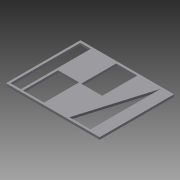
# Autodesk Inventor part: Molecule Chopper
Saved by Autodesk Inventor 2015 (Build 190159000, 159)
## iProperties
Created: 2014-07-07
Part Number: Molecule Chopper
Material: Generic
Document SubType Name: Modeling
Designer: I Rabey
Density: 1 g/cm^3
Appearance: Default
Author: I Rabey
Autodesk Inventor part; units mm, degrees
ref_plane "YZ Plane" through (0, 0, 0) normal (1, 0, 0) x (0, 1, 0)
ref_plane "XZ Plane" through (0, 0, 0) normal (0, 1, 0) x (-1, 0, 0)
ref_plane "XY Plane" through (0, 0, 0) normal (0, 0, 1) x (1, 0, 0)
sketch "Sketch1" plane through (0, 0, 0) normal (0, 1, 0) x (-1, 0, 0)
  line L0 (-42.5, 33.75) -> (42.5, 33.75)
  line L1 (42.5, 33.75) -> (42.5, -33.75)
  line L2 (42.5, -33.75) -> (-42.5, -33.75)
  line L3 (-42.5, -33.75) -> (-42.5, 33.75)
  line L4 (-42.5, 33.75) -> (42.5, -33.75) construction
  line L5 (42.5, 33.75) -> (-42.5, -33.75) construction
  line L6 (60.5225, 31.75) -> (41.4725, 31.75)
  line L7 (40.5, 31.75) -> (30.9975, 31.75)
  line L8 (30.9975, 31.75) -> (30.9975, -31.75)
  line L9 (30.9975, -31.75) -> (40.5, -31.75)
  line L10 (40.5, -31.75) -> (40.5, 31.75)
  line L11 (40.5, 31.75) -> (30.9975, -31.75) construction
  line L12 (30.9975, 31.75) -> (40.5, -31.75) construction
  line L13 (28.9975, 31.75) -> (9.9475, 31.75)
  line L14 (9.9475, 31.75) -> (9.9475, 0)
  line L15 (9.9475, 0) -> (28.9975, 0)
  line L16 (28.9975, 0) -> (28.9975, 31.75)
  line L17 (7.9475, 0) -> (-11.1025, 0)
  line L18 (-11.1025, 0) -> (-11.1025, -31.75)
  line L19 (-11.1025, -31.75) -> (7.9475, -31.75)
  line L20 (7.9475, -31.75) -> (7.9475, 0)
  line L21 (-13.1025, 31.75) -> (-32.1525, 31.75)
  line L22 (-32.1525, 31.75) -> (-32.1525, -31.75)
  line L23 (-32.1525, -31.75) -> (-13.1025, 31.75)
  point P0 (0, 0)
  point P1 (35.7488, 0)
  dimension "d0" = 85
  dimension "d1" = 67.5
  dimension "d5" = 9.5025
  dimension "d6" = 63.5
  dimension "d9" = 19.05
  dimension "d10" = 31.75
  dimension "d11" = 0
  dimension "d12" = 2
  dimension "d13" = 19.05
  dimension "d14" = 31.75
  dimension "d15" = 0
  dimension "d16" = 2
  dimension "d17" = 19.05
  dimension "d19" = 0
  dimension "d20" = 2
  dimension "d26" = 2
  dimension "d30" = 10.3475
  constraints: 48 end point, 8 parallel, 6 horizontal, 5 perpendicular, 4 midpoint
  measures "d0" distance of L1.end L2.end
  measures "d1" distance of L0.end L1.end
  measures "d5" distance of L9.end L8.end
  measures "d6" distance of L8.end L7.end
  measures "d9" distance of L15.end L14.end
  measures "d10" distance of L14.end L13.end
  measures "d11" vertical distance of L13.start L7.end
  measures "d12" distance between parallel lines of L8 L16
  measures "d13" distance of L19.end L18.end
  measures "d14" distance of L18.end L17.end
  measures "d15" vertical distance of L8.end L19.end
  measures "d16" distance between parallel lines of L14 L20
  measures "d17" distance of L21.start L21.end
  measures "d19" vertical distance of L21.start L13.end
  measures "d20" horizontal distance of L17.end L21.start
  measures "d26" distance between parallel lines of L1 L10
  measures "d30" distance between parallel lines of L3 L22
extrude "Extrusion3" add sketch "Sketch1" along normal blind 2
body "Solid3"
